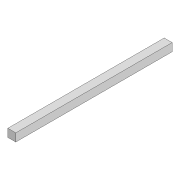
# Autodesk Inventor part: Träger Seiten
Saved by Autodesk Inventor 2020 (Build 240168000, 168)
## iProperties
Created: 2021-06-23
Part Number: Träger Seiten
Material: Generisch
Document SubType Name: Modeling
Designer: mike8
Density: 1 g/cm^3
Appearance: Vorgabe
Author: mike8
Autodesk Inventor part; units mm, degrees
ref_plane "YZ Plane" through (0, 0, 0) normal (1, 0, 0) x (0, 1, 0)
ref_plane "XZ Plane" through (0, 0, 0) normal (0, 1, 0) x (-1, 0, 0)
ref_plane "XY Plane" through (0, 0, 0) normal (0, 0, 1) x (1, 0, 0)
sketch "Skizze1" plane through (0, 0, 0) normal (0, 0, 1) x (1, 0, 0)
  line L0 (-24.4513, 0) -> (17.5487, 0) projected
  line L1 (0, -18.8761) -> (0, 23.1239) projected
  line L2 (11.5487, -12.8761) -> (-18.4513, -12.8761)
  line L3 (-18.4513, -12.8761) -> (-18.4513, 17.1239)
  line L4 (-18.4513, 17.1239) -> (11.5487, 17.1239)
  line L5 (11.5487, 17.1239) -> (11.5487, -12.8761)
  point P0 (0, 0)
  dimension "d0" = 30
  dimension "d1" = 30
  constraints: 8 end point, 2 parallel, 1 horizontal, 1 perpendicular
  measures "d0" distance of L3.end L4.end
  measures "d1" distance of L4.end L2.start
extrude "Extrusion1" add sketch "Skizze1" along normal blind 590
